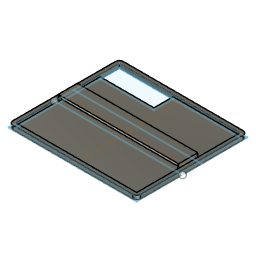
Center Side Up Cover 1x1 v3 (Autodesk Fusion 360 design; units mm, degrees)
Autodesk Fusion 360 part; units mm, degrees
sketch "Schizzo1" plane through (0, 0, 0) normal (0, 0, 1) x (1, 0, 0)
  line L0 (15, 63.85) -> (81.7, 63.85) construction
  line L1 (81.7, 63.85) -> (81.7, 6.15) construction
  line L2 (81.7, 6.15) -> (15, 6.15) construction
  line L3 (15, 6.15) -> (15, 63.85) construction
  line L4 (15, 35) -> (81.7, 35) construction
  line L5 (48.35, 63.85) -> (48.35, 6.15) construction
  line L6 (81.6, 6.25) -> (15.1, 6.25)
  line L7 (15.1, 6.25) -> (15.1, 63.75)
  line L8 (15.1, 63.75) -> (81.6, 63.75)
  line L9 (81.6, 63.75) -> (81.6, 6.25)
  line L10 (79.7, 8.15) -> (17, 8.15)
  line L11 (17, 8.15) -> (17, 61.85)
  line L12 (17, 61.85) -> (79.7, 61.85)
  line L13 (79.7, 61.85) -> (79.7, 8.15)
  line L14 (15.1, 40) -> (81.7, 40)
  line L15 (15.1, 30) -> (81.7, 30)
  line L16 (17, 61.85) -> (45, 61.85)
  line L17 (45, 61.85) -> (45, 51.85)
  line L18 (45, 51.85) -> (17, 51.85)
  line L19 (17, 51.85) -> (17, 61.85)
  dimension "d1" = 66.7
  dimension "d2" = 57.7
  dimension "d3" = 0.1
  dimension "d4" = 2
  dimension "d9" = 10
  dimension "d18" = 28
  dimension "d19" = 10
  constraint horizontal L0
  constraint vertical L1
  constraint horizontal L2
  constraint vertical L3
  constraint coincident L3 L4.start
  constraint coincident L1 L4.end
  constraint perpendicular L1 L4
  constraint midpoint L3 L4.start
  constraint midpoint L0 L5.start
  constraint midpoint L2 L5.end
  constraint coincident L7 L14.start
  constraint coincident L1 L14.end
  constraint perpendicular L1 L14
  constraint symmetric L4 L14.start L15.start
  constraint symmetric L4 L14.end L15.end
  constraint horizontal L16
  constraint vertical L17
  constraint horizontal L18
  constraint vertical L19
  measures "d1" distance of L0.start L0.end
  measures "d2" distance of L0.start L2.end
  measures "d9" distance of L14 L15
  measures "d18" distance of L11.end L16.end
  measures "d19" distance of L11.end L18.end
extrude "Estrusione1" add sketch "Schizzo1" along normal blind 1 contours L11 L13 L14 L15 | L10 L11 L13 L15 | L11 L12 L13 L14 L17 L18
extrude "Estrusione2" add sketch "Schizzo1" along normal blind 2 contours L6 L7 L9 L10 L11 L13 L15 | L9 L13 L14 L15 | L7 L11 L14 L15 | L7 L8 L9 L11 L12 L13 L14 L16 L19
fillet "Raccordo1" radius 2 4 edges at (81.6, 6.25, 1) (15.1, 6.25, 1) (81.6, 63.75, 1) (15.1, 63.75, 1)
extrude "Estrusione3" add sketch "Schizzo1" along normal blind 4 contours L11 L13 L14 L15
ref_plane "Piano di lavoro1" through (48.35, 35, 0) normal (-1, 0, 0) x (0, -1, 0)
sketch "Schizzo2" plane through (48.35, 0, 0) normal (-1, 0, 0) x (0, -1, 0)
  line L0 (-30, 4) -> (-40, 4) construction
  line L1 (-40, 4) -> (-40, 1) construction
  line L2 (-40, 1) -> (-30, 1) construction
  line L3 (-30, 1) -> (-30, 4) construction
  line L4 (-30, 1) -> (-30, 4)
  line L5 (-30, 4) -> (-31.7321, 1)
  line L6 (-31.7321, 1) -> (-30, 1)
  line L7 (-35, 4) -> (-35, 1) construction
  line L8 (-40, 4) -> (-38.2679, 1)
  line L9 (-40, 1) -> (-40, 4) construction
  line L10 (-38.2679, 1) -> (-40, 1)
  line L11 (-40, 1) -> (-40, 4)
  point P0 (-40, 1)
  point P1 (-30, 4)
  dimension "d15" = 30
  constraint horizontal L0
  constraint vertical L1
  constraint horizontal L2
  constraint vertical L3
  constraint coincident P0 L1.end
  constraint coincident L0.start L3.end
  constraint coincident L2 L5.end
  constraint midpoint L0 L7.start
  constraint midpoint L2 L7.end
  constraint symmetric L0.start L7 L0.end
  constraint symmetric L2.end L7 P0
  constraint symmetric L5.end L7 L8.end
  measures "d15" angle of L4 L5
extrude "Estrusione4" cut sketch "Schizzo2" along normal mid plane 62
